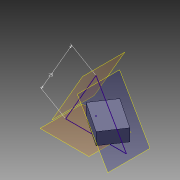
# Autodesk Inventor part: fit_test
Saved by Autodesk Inventor 2014 SP1 (Build 180222100, 222)
## iProperties
Created: 2014-11-10
Part Number: fit_test
Material: Generic
Document SubType Name: Modeling
Designer: rawrdong
Density: 1 g/cm^3
Appearance: Default
Author: rawrdong
Autodesk Inventor part; units mm, degrees
ref_plane "YZ Plane" through (0, 0, 0) normal (1, 0, 0) x (0, 1, 0)
ref_plane "XY Plane" through (0, 0, 0) normal (0, 0, 1) x (1, 0, 0)
sketch "Sketch1" plane through (0, 0, 0) normal (0, 1, 0) x (-1, 0, 0)
  line L0 (0, 14.4338) -> (12.5, -7.2169)
  line L1 (12.5, -7.2169) -> (-12.5, -7.2169)
  line L2 (-12.5, -7.2169) -> (0, 14.4338)
  point P0 (0, 0)
  point P1 (0, 0)
  dimension "d7" = 25
  constraints: 6 end point, 1 coincident, 1 vertical alignment, 7 other
  measures "d7" distance of L0.start L0.end
ref_plane "Work Plane1" through (0, 0, 14.4338) normal (0.866, 0, -0.5) x (-0.5, 0, -0.866)
ref_plane "Work Plane2" through (12.5, 0, -7.2169) normal (-0.866, 0, -0.5) x (-0.5, 0, 0.866)
ref_plane "Work Plane3" through (-12.5, 0, -7.2169) normal (0, 0, 1) x (1, 0, 0)
sketch "Sketch2" plane through (-12.5, 0, -7.2169) normal (0, 0, 1) x (1, 0, 0)
  line L0 (15.9537, -3.3702) -> (3.4861, 4.97)
  line L1 (3.4861, 4.97) -> (9.0463, 13.2818)
  line L2 (9.0463, 13.2818) -> (21.5139, 4.9416)
  line L3 (21.5139, 4.9416) -> (15.9537, -3.3702)
  line L4 (15.9537, -3.3702) -> (9.0463, 13.2818) construction
  line L5 (3.4861, 4.97) -> (21.5139, 4.9416) construction
  point P0 (12.5, 0)
  point P1 (12.5, 4.9558)
  point P2 (12.5, 4.9558)
  dimension "d3" = 15
  dimension "d4" = 10
  constraints: 12 end point, 3 midpoint, 2 parallel, 1 perpendicular, 1 vertical alignment
  measures "d3" distance of L0.start L0.end
  measures "d4" distance of L0.end L1.end
extrude "Extrusion1" add sketch "Sketch2" along normal blind 5
body "Solid1"
